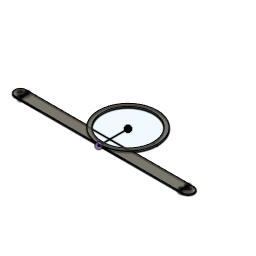
respirator-strap v15 v4 (Autodesk Fusion 360 design; units mm, degrees)
Autodesk Fusion 360 part; units mm, degrees
sketch "Sketch1" plane through (0, 0, 0) normal (0, 1, 0) x (1, 0, 0) in component "strap"
  circle A0 centre (0, 40) radius 35
  line L0 (0, 0) -> (0, 40)
  circle A1 centre (0, 40) radius 40
  line L1 (115, 15) -> (0, 15)
  line L2 (0, 0) -> (115, 0)
  line L3 (0, 15) -> (-115, 15)
  line L4 (-115, 0) -> (0, 0)
  arc A2 (-115, 15) -> (-115, 0) centre (-115, 7.5) ccw
  arc A3 (115, 0) -> (115, 15) centre (115, 7.5) ccw
  line L5 (-111, 12) -> (-111, 3)
  arc A4 (-111, 3) -> (-109, 3) centre (-110, 3) ccw
  line L6 (-109, 3) -> (-109, 12)
  arc A5 (-109, 12) -> (-111, 12) centre (-110, 12) ccw
  line L7 (-110, 13) -> (-110, 2) construction
  line L8 (109, 3) -> (109, 12)
  line L9 (111, 12) -> (111, 3)
  arc A6 (109, 3) -> (111, 3) centre (110, 3) ccw
  arc A7 (111, 12) -> (109, 12) centre (110, 12) ccw
  dimension "d1" = 70
  dimension "d2" = 40
  dimension "d3" = 80
  dimension "d55" = 115
  dimension "d56" = 115
  dimension "d57" = 15
  dimension "d58" = 2
  dimension "d59" = 3
  dimension "d60" = 3
  dimension "d61" = 110
  constraint vertical L0
  constraint coincident A0.centre L0.end
  constraint concentric A0 A1
  constraint coincident L0.start A1
  constraint horizontal L1
  constraint coincident L0.start L2.start
  constraint coincident L0 L1.end
  constraint tangent A1 L2
  constraint parallel L1 L3
  constraint tangent L4 A2
  constraint tangent L3 A2
  constraint tangent L2 A3
  constraint tangent L1 A3
  constraint horizontal L4
  constraint tangent L5 A4
  constraint tangent A4 L6
  constraint parallel L5 L6
  constraint tangent L6 A5
  constraint tangent L5 A5
  constraint midpoint A5 L7.start
  constraint midpoint A4 L7.end
  constraint vertical L7
  constraint symmetric L0 L5.start L9.start
  constraint symmetric L0 L5.end L9.end
  constraint symmetric L0 A4.end L8.start
  constraint symmetric L0 L6.end L8.end
  constraint symmetric L0 A4 A6
  constraint symmetric L0 A5 A7
  measures "d1" diameter of A0
  measures "d2" distance of L0.start A0.centre
  measures "d3" diameter of A1
  measures "d55" distance of L4.start L0.start
  measures "d56" distance of L0.start L2.end
  measures "d57" distance of L3 L4
  measures "d58" diameter of A4
  measures "d59" distance of L3 A5.centre
  measures "d60" distance of L4 A4.centre
  measures "d61" horizontal distance of L0.start A4.centre
extrude "Extrude4" add sketch "Sketch1" along normal blind 2 contours A0 A1 L1 L3 | A0 L0 A1 L3 | A0 L0 A1 L1 makes body 1 in component "strap"
extrude "Extrude5" add sketch "Sketch1" along normal blind 1.5 contours A1 L3 L4 A2 | A1 L1 L2 A3 bodies 1 in component "strap"
extrude "Extrude2" [rolled back] along distance 1.5 taper angle 0
sketch "Sketch3" plane through (0, 0, 0) normal (0, 1, 0) x (1, 0, 0) in component "strap"
  line L0 (0, 0) -> (200, 0) construction
  line L1 (190, 0) -> (190, -5)
  line L2 (190, 0) -> (190, 5)
  line L3 (150, 0) -> (150, 20)
  line L4 (150, 0) -> (150, -20)
  line L5 (80, 0) -> (80, 60)
  line L6 (80, 0) -> (80, -60)
  spline S0 degree 5 poles (0, 50) (2.5133, 51.6602) (7.5371, 54.7649) (15.0646, 58.7751) (25.0847, 62.827) (37.5784, 65.7422) (50.0287, 66.5474) (62.4121, 65.3317) (74.6891, 62.2543) (86.8014, 57.5606) (98.6648, 51.6107) (110.1782, 44.8596) (121.2442, 37.7974) (131.7861, 30.9026) (141.7679, 24.5888) (151.2098, 19.1563) (160.214, 14.7361) (168.9636, 11.2501) (177.5638, 8.4909) (185.8694, 6.1929) (193.3726, 4.1001) (198.9302, 2.0512) (201.0437, 0) (198.9302, -2.0512) (193.3726, -4.1001) (185.8694, -6.1929) (177.5638, -8.4909) (168.9636, -11.2501) (160.214, -14.7361) (151.2098, -19.1563) (141.7679, -24.5888) (131.7861, -30.9026) (121.2442, -37.7974) (110.1782, -44.8596) (98.6648, -51.6107) (86.8014, -57.5606) (74.6891, -62.2543) (62.4121, -65.3317) (50.0287, -66.5474) (37.5784, -65.7422) (25.0847, -62.827) (15.0646, -58.7751) (7.5371, -54.7649) (2.5133, -51.6602) (0, -50) knots 0 0 0 0 0 0 0.025 0.05 0.075 0.1 0.125 0.15 0.175 0.2 0.225 0.25 0.275 0.3 0.325 0.35 0.375 0.4 0.425 0.45 0.475 0.5 0.525 0.55 0.575 0.6 0.625 0.65 0.675 0.7 0.725 0.75 0.775 0.8 0.825 0.85 0.875 0.9 0.925 0.95 0.975 1 1 1 1 1 1
  line L7 (0, 50) -> (0, -50)
  point P0 (0, 50)
  point P1 (0, -50)
  dimension "d14" = 200
  dimension "d15" = 5
  dimension "d16" = 5
  dimension "d17" = 10
  dimension "d18" = 20
  dimension "d19" = 20
  dimension "d20" = 60
  dimension "d21" = 60
  dimension "d22" = 50
  dimension "d23" = 120
  dimension "d40" = 50
  dimension "d41" = 50
  constraint coincident L0.start origin
  constraint horizontal L0
  constraint coincident L0 L1.start
  constraint perpendicular L0 L1
  constraint perpendicular L0 L2
  constraint coincident L0 L3.start
  constraint perpendicular L0 L3
  constraint perpendicular L0 L4
  constraint coincident L0 L5.start
  constraint perpendicular L0 L5
  constraint perpendicular L0 L6
  constraint coincident P0 S0.start
  constraint coincident P1 S0.end
  constraint vertical L7
  constraint coincident L0.start L7
  measures "d14" distance of L0.start L0.end
  measures "d15" distance of L1.start L1.end
  measures "d16" distance of L1.start L2.end
  measures "d17" distance of L0.end L2
  measures "d18" distance of L3.start L3.end
  measures "d19" distance of L3.start L4.end
  measures "d20" distance of L5.start L5.end
  measures "d21" distance of L5.start L6.end
  measures "d22" distance of L0.end L3
  measures "d23" distance of L0.end L5
  measures "d40" distance of L0 P0
  measures "d41" distance of L0 P1
ref_plane "WorkPlane3" through (0, 12, 0) normal (0, 1, 0) x (0, 0, 1) in component "strap"
sketch "Sketch4" plane through (0, 12, 0) normal (0, 1, 0) x (1, 0, 0) in component "strap"
  line L0 (0, 0) -> (210, 0)
  line L1 (195, 7) -> (195, -7)
  line L2 (150, 40) -> (150, -40)
  line L3 (77, 60) -> (77, -60)
  spline S0 degree 5 poles (0, 50) (2.2239, 50.65) (6.7292, 51.9004) (13.6596, 53.627) (23.2451, 55.6305) (35.7897, 57.6281) (48.856, 59.0937) (62.3594, 59.979) (76.1556, 60.2056) (90.0263, 59.6581) (103.6602, 58.1747) (116.7139, 55.5905) (128.8769, 51.7838) (139.9352, 46.7209) (149.8374, 40.503) (158.7558, 33.4106) (167.1624, 25.9558) (175.5914, 18.7589) (184.4, 12.4211) (193.5076, 7.3938) (202.1937, 3.86) (208.7335, 1.5796) (211.2344, 0) (208.7335, -1.5796) (202.1937, -3.86) (193.5076, -7.3938) (184.4, -12.4211) (175.5914, -18.7589) (167.1624, -25.9558) (158.7558, -33.4106) (149.8374, -40.503) (139.9352, -46.7209) (128.8769, -51.7838) (116.7139, -55.5905) (103.6602, -58.1747) (90.0263, -59.6581) (76.1556, -60.2056) (62.3594, -59.979) (48.856, -59.0937) (35.7897, -57.6281) (23.2451, -55.6305) (13.6596, -53.627) (6.7292, -51.9004) (2.2239, -50.65) (0, -50) knots 0 0 0 0 0 0 0.025 0.05 0.075 0.1 0.125 0.15 0.175 0.2 0.225 0.25 0.275 0.3 0.325 0.35 0.375 0.4 0.425 0.45 0.475 0.5 0.525 0.55 0.575 0.6 0.625 0.65 0.675 0.7 0.725 0.75 0.775 0.8 0.825 0.85 0.875 0.9 0.925 0.95 0.975 1 1 1 1 1 1
  line L4 (0, 50) -> (0, -50)
  point P0 (0, 50)
  point P1 (0, -50)
  dimension "d29" = 210
  dimension "d31" = 15
  dimension "d32" = 60
  dimension "d33" = 133
  dimension "d34" = 60
  dimension "d35" = 60
  dimension "d36" = 40
  dimension "d37" = 40
  dimension "d38" = 7
  dimension "d39" = 7
  constraint coincident L0.start origin
  constraint horizontal L0
  constraint perpendicular L0 L1
  constraint perpendicular L0 L2
  constraint perpendicular L0 L3
  constraint coincident P0 S0.start
  constraint coincident P1 S0.end
  measures "d29" distance of L0.start L0.end
  measures "d31" distance of L0.end L1
  measures "d32" distance of L0.end L2
  measures "d33" distance of L0.end L3
  measures "d34" distance of L0 L3.start
  measures "d35" distance of L0 L3.end
  measures "d36" distance of L0 L2.start
  measures "d37" distance of L0 L2.end
  measures "d38" distance of L0 L1.start
  measures "d39" distance of L0 L1.end
form_body "Form1" makes body 2 makes body 3 in component "strap"
extrude "Extrude1" [rolled back] along distance 2 taper angle 0 in component "strap"
extrude "Extrude2'" [rolled back] along distance 9.478 taper angle 0 against distance 8.698 side2taper angle 0 in component "strap"
extrude "Extrude3" [rolled back] along distance 8.481 taper angle 0 in component "strap"
component "strap" placed x (1, 0, 0) y (0, 1, 0) z (0, 0, 1) at (0, 0, 0)
